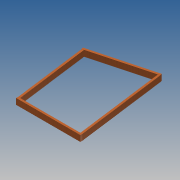
# Autodesk Inventor part: panelDframe
Saved by Autodesk Inventor 2014 SP1 (Build 180222100, 222)
## iProperties
Created: 2015-04-29
Part Number: panelDframe
Material: Wood (Cherry)
Document SubType Name: Modeling
Designer: Dave
Mass: 15299.2 g
Surface Area: 17040 cm^2
Volume: 24284.5 cm^3
Density: 0.63 g/cm^3
Appearance: Cherry - Natural Low Gloss
Author: Dave
Autodesk Inventor part; units mm, degrees
ref_plane "YZ Plane" through (0, 0, 0) normal (1, 0, 0) x (0, 1, 0)
ref_plane "XZ Plane" through (0, 0, 0) normal (0, 1, 0) x (-1, 0, 0)
ref_plane "XY Plane" through (0, 0, 0) normal (0, 0, 1) x (1, 0, 0)
sketch "Sketch1" plane through (0, 0, 0) normal (0, 1, 0) x (-1, 0, 0)
  line L0 (-988.9153, -1793.2204) -> (194.3412, -1476.1678)
  line L1 (189.3384, -1438.1678) -> (5.0028, -38)
  line L2 (-998.7504, -1756.5152) -> (-1225.2435, -36.1295)
  line L3 (-961.7285, -1746.5952) -> (152.3165, -1448.0878)
  line L4 (152.3165, -1448.0878) -> (-33.3251, -38)
  line L5 (-33.3251, -38) -> (-1186.6693, -38)
  line L6 (-961.7285, -1746.5952) -> (-1186.6693, -38)
  line L7 (-998.7504, -1756.5152) -> (-988.9153, -1793.2204)
  line L8 (-1225.2435, -36.1295) -> (-1225.2435, 0)
  line L9 (189.3384, -1438.1678) -> (199.1735, -1474.873)
  line L10 (194.3412, -1476.1678) -> (199.1735, -1474.873)
  line L11 (5.0028, -38) -> (5.0028, 0)
  line L12 (5.0028, 0) -> (-1225.2435, 0)
  dimension "d7" = 38
  dimension "d8" = 38
  constraints: 26 end point, 3 perpendicular, 2 parallel
  measures "d7" distance between parallel lines of L3 L0
  measures "d8" distance between parallel lines of L2 L6
extrude "Extrusion1" add sketch "Sketch1" along normal blind 114
sketch "Sketch2" plane through (0, 114, 0) normal (0, 1, 0) x (1, 0, 0)
  line L0 (33.3251, 38) -> (-152.3165, 1448.0878) projected
  line L1 (-189.3384, 1438.1678) -> (-5.0028, 38) projected
  line L2 (-5.0028, 38) -> (-5.0028, 0) projected
  line L3 (998.7504, 1756.5152) -> (988.9153, 1793.2204) projected
  line L4 (-152.3165, 1448.0878) -> (-189.3384, 1438.1678)
  line L5 (33.3251, 38) -> (-5.0028, 38)
  point P0 (0, 0)
  constraints: 4 end point, 2 perpendicular
extrude "Extrusion2" cut sketch "Sketch2" against normal blind 1
sketch "Sketch4" plane through (0, 114, 0) normal (0, 1, 0) x (1, 0, 0)
  line L0 (961.7285, 1746.5952) -> (1186.6693, 38) projected
  line L1 (1225.2435, 0) -> (1225.2435, 36.1295) projected
  line L2 (1225.2435, 36.1295) -> (998.7504, 1756.5152) projected
  line L3 (-199.1735, 1474.873) -> (-189.3384, 1438.1678) projected
  line L4 (961.7285, 1746.5952) -> (998.7504, 1756.5152)
  line L5 (1186.6693, 38) -> (1224.9972, 38)
  point P0 (0, 0)
  constraints: 4 end point, 2 perpendicular, 1 point on line
extrude "Extrusion4" cut sketch "Sketch4" against normal blind 1
body "Solid1"
